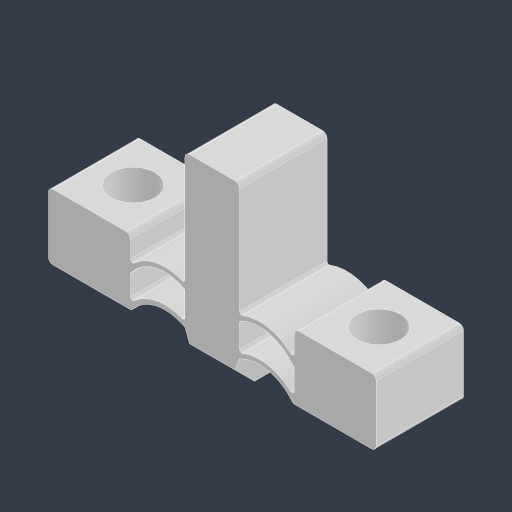
# Autodesk Inventor part: Actuator
Saved by Autodesk Inventor 2023.4 (Build 274418000, 418)
## iProperties
Created: 2024-02-27
Part Number: Actuator
Material: Generic
Document SubType Name: Modeling
Designer: JoaoSilva
Density: 1 g/cm^3
Appearance: Default
Author: JoaoSilva
Autodesk Inventor part; units mm, degrees
ref_plane "YZ Plane" through (0, 0, 0) normal (1, 0, 0) x (0, 1, 0)
ref_plane "XZ Plane" through (0, 0, 0) normal (0, 1, 0) x (-1, 0, 0)
ref_plane "XY Plane" through (0, 0, 0) normal (0, 0, 1) x (1, 0, 0)
sketch "Sketch1" plane through (0, 0, 0) normal (0, 0, 1) x (1, 0, 0)
  line L0 (-2.5, 9) -> (2.5, 9)
  line L1 (2.5, 9) -> (2.5, -9)
  line L2 (2.5, -9) -> (-2.5, -9)
  line L3 (-2.5, -9) -> (-2.5, 9)
  line L4 (-2.5, 9) -> (2.5, -9) construction
  line L5 (2.5, 9) -> (-2.5, -9) construction
  line L6 (-15, 0) -> (-7.5, 0)
  line L7 (-7.5, 0) -> (-7.5, -3)
  line L8 (-7.5, -3) -> (-15, -3)
  line L9 (-15, -3) -> (-15, 0)
  line L10 (7.5, 0) -> (15, 0)
  line L11 (15, 0) -> (15, -3)
  line L12 (15, -3) -> (7.5, -3)
  line L13 (7.5, -3) -> (7.5, 0)
  line L14 (7.5, -3) -> (7.5, -6)
  line L15 (7.5, -6) -> (15, -6)
  line L16 (15, -6) -> (15, -3)
  line L17 (-7.5, -3) -> (-7.5, -6)
  line L18 (-7.5, -6) -> (-15, -6)
  line L19 (-15, -6) -> (-15, -3)
  line L20 (-7.5, -1.5) -> (7.5, -1.5) construction
  line L21 (-1, -9) -> (-2.5, -4.878784)
  line L22 (1, -9) -> (2.5, -4.878784)
  arc A0 (-2.5, -4.678784) -> (-7.5, -5.8) centre (-4.32787, -8.236717) ccw construction
  arc A1 (-2.408606, -4.500887) -> (-7.658606, -5.678164) centre (-4.32787, -8.236717) ccw
  arc A2 (-2.591394, -4.856681) -> (-7.341394, -5.921836) centre (-4.32787, -8.236717) ccw
  arc A3 (-2.591394, -4.856681) -> (-2.408606, -4.500887) centre (-2.5, -4.678784) ccw
  arc A4 (-7.658606, -5.678164) -> (-7.341394, -5.921836) centre (-7.5, -5.8) ccw
  arc A5 (7.5, -5.8) -> (2.5, -4.678784) centre (4.32787, -8.236717) ccw construction
  arc A6 (7.658606, -5.678164) -> (2.408606, -4.500887) centre (4.32787, -8.236717) ccw
  arc A7 (7.341394, -5.921836) -> (2.591394, -4.856681) centre (4.32787, -8.236717) ccw
  arc A8 (7.341394, -5.921836) -> (7.658606, -5.678164) centre (7.5, -5.8) ccw
  arc A9 (2.408606, -4.500887) -> (2.591394, -4.856681) centre (2.5, -4.678784) ccw
  arc A10 (-2.5, -1.678784) -> (-7.5, -2.8) centre (-4.32787, -5.236717) ccw construction
  arc A11 (-2.408606, -1.500887) -> (-7.658606, -2.678164) centre (-4.32787, -5.236717) ccw
  arc A12 (-2.591394, -1.856681) -> (-7.341394, -2.921836) centre (-4.32787, -5.236717) ccw
  arc A13 (-2.591394, -1.856681) -> (-2.408606, -1.500887) centre (-2.5, -1.678784) ccw
  arc A14 (-7.658606, -2.678164) -> (-7.341394, -2.921836) centre (-7.5, -2.8) ccw
  arc A15 (7.5, -2.8) -> (2.5, -1.678784) centre (4.32787, -5.236717) ccw construction
  arc A16 (7.658606, -2.678164) -> (2.408606, -1.500887) centre (4.32787, -5.236717) ccw
  arc A17 (7.341394, -2.921836) -> (2.591394, -1.856681) centre (4.32787, -5.236717) ccw
  arc A18 (7.341394, -2.921836) -> (7.658606, -2.678164) centre (7.5, -2.8) ccw
  arc A19 (2.408606, -1.500887) -> (2.591394, -1.856681) centre (2.5, -1.678784) ccw
  point P0 (0, 0)
  point P1 (0, -1.5)
  point P2 (-7.5, -5.483975)
  point P3 (-2.5, -1.878784)
  point P4 (-2.5, -4.45533)
  point P5 (7.5, -5.483975)
  point P6 (2.5, -4.45533)
  point P7 (2.5, -1.878784)
  point P8 (7.5, -2.483975)
  point P9 (2.5, -1.45533)
  point P10 (-2.5, -1.45533)
  point P11 (-7.5, -2.483975)
  dimension "d0" = 5
  dimension "d1" = 18
  dimension "d2" = 30
  dimension "d3" = 3
  dimension "d4" = 3
  dimension "d5" = 5
  dimension "d8" = 9
  dimension "d9" = 3
  dimension "d10" = 2
  dimension "d11" = 20
  dimension "d12" = 0.4
  dimension "d13" = 4
  dimension "d14" = 3
  constraints: 46 end point, 42 point on circle, 20 centre point, 18 tangent, 14 point on line, 7 perpendicular, 6 equal radius, 6 parallel, 5 midpoint, 3 collinear, 3 equal length, 3 horizontal, 3 vertical alignment, 2 horizontal alignment, 2 vertical
  measures "d0" distance of L0.start L0.end
  measures "d1" distance of L0.end L1.end
  measures "d2" distance between parallel lines of L11 L9
  measures "d3" distance between parallel lines of L2 L18
  measures "d4" distance between parallel lines of L2 L15
  measures "d5" distance between parallel lines of L3 L17
  measures "d8" distance between parallel lines of L2 L6
  measures "d9" distance of L8.end L6.start
  measures "d10" distance of L22.start L21.start
  measures "d11" angle of L3 L21
  measures "d12" radial gap between concentric circles of A1 A2
  measures "d13" radius of A0
  measures "d14" distance of A0.centre A10.centre
sketch "Sketch1 outline for Extrusion1" plane through (0, 0, 0) normal (0, 0, 1) x (1, 0, 0)
  arc A0 (-7.5, -6) -> (-7.341394, -5.921836) centre (-7.5, -5.8) ccw
  line L0 (-15, -6) -> (-7.5, -6)
  arc A1 (-7.341394, -5.921836) -> (-2.591394, -4.856681) centre (-4.32787, -8.236717) cw
  line L1 (-15, -3) -> (-15, -6)
  arc A2 (-2.591394, -4.856681) -> (-2.5, -4.878784) centre (-2.5, -4.678784) ccw
  line L2 (-15, 0) -> (-15, -3)
  line L3 (-2.5, -4.878784) -> (-1, -9)
  line L4 (-7.5, 0) -> (-15, 0)
  line L5 (-1, -9) -> (1, -9)
  line L6 (-7.5, -2.483975) -> (-7.5, 0)
  line L7 (1, -9) -> (2.5, -4.878784)
  arc A3 (-2.5, -1.45533) -> (-7.5, -2.483975) centre (-4.32787, -5.236717) ccw
  arc A4 (2.5, -4.878784) -> (2.591394, -4.856681) centre (2.5, -4.678784) ccw
  line L8 (-2.5, 9) -> (-2.5, -1.45533)
  arc A5 (2.591394, -4.856681) -> (7.341394, -5.921836) centre (4.32787, -8.236717) cw
  line L9 (2.5, 9) -> (-2.5, 9)
  arc A6 (7.341394, -5.921836) -> (7.5, -6) centre (7.5, -5.8) ccw
  line L10 (2.5, -1.45533) -> (2.5, 9)
  line L11 (7.5, -6) -> (15, -6)
  arc A7 (7.5, -2.483975) -> (2.5, -1.45533) centre (4.32787, -5.236717) ccw
  line L12 (15, -6) -> (15, -3)
  line L13 (7.5, 0) -> (7.5, -2.483975)
  line L14 (15, -3) -> (15, 0)
  line L15 (15, 0) -> (7.5, 0)
  line L16 (-7.5, -5.483975) -> (-7.5, -3)
  arc A8 (-2.5, -4.45533) -> (-7.5, -5.483975) centre (-4.32787, -8.236717) ccw
  line L17 (-2.5, -1.878784) -> (-2.5, -4.45533)
  arc A9 (-2.591394, -1.856681) -> (-2.5, -1.878784) centre (-2.5, -1.678784) ccw
  arc A10 (-7.341394, -2.921836) -> (-2.591394, -1.856681) centre (-4.32787, -5.236717) cw
  arc A11 (-7.5, -3) -> (-7.341394, -2.921836) centre (-7.5, -2.8) ccw
  arc A12 (7.5, -5.483975) -> (2.5, -4.45533) centre (4.32787, -8.236717) ccw
  line L18 (7.5, -3) -> (7.5, -5.483975)
  arc A13 (7.341394, -2.921836) -> (7.5, -3) centre (7.5, -2.8) ccw
  arc A14 (2.591394, -1.856681) -> (7.341394, -2.921836) centre (4.32787, -5.236717) cw
  arc A15 (2.5, -1.878784) -> (2.591394, -1.856681) centre (2.5, -1.678784) ccw
  line L19 (2.5, -4.45533) -> (2.5, -1.878784)
extrude "Extrusion1" add sketch "Sketch1 outline for Extrusion1" along normal blind 8
chamfer "Chamfer1" distance 3 angle 45 1 edges at (0, -9, 0) measured on face at (-0.3333, -9, 2.6667)
chamfer "Chamfer2" distance 3 angle 45 1 edges at (0, -9, 8) measured on face at (-0.3333, -9, 4.6667)
fillet "Fillet1" radius 0.2 14 edges at (-7.5, -2.484, 4) (-7.5, -3, 4) (-7.5, -5.484, 4) (-2.5, -4.8788, 4) (-2.5, -4.4553, 4) (-2.5, -1.8788, 4) (-2.5, -1.4553, 4) (2.5, -1.4553, 4) (2.5, -1.8788, 4) (2.5, -4.4553, 4) (2.5, -4.8788, 4) (7.5, -5.484, 4) (7.5, -3, 4) (7.5, -2.484, 4)
fillet "Fillet2" radius 0.4 12 edges at (-15, 0, 4) (-15, -3, 4) (15, -3, 4) (15, 0, 4) (7.5, 0, 4) (15, -6, 4) (-15, -6, 4) (-7.5, 0, 4) (-2.5, 9, 4) (2.5, 9, 4) (-1, -9, 4) (1, -9, 4)
sketch "Sketch3" plane through (-14.6, 0, 0) normal (0, 1, 0) x (1, 0, 0)
  line L0 (3.35, -4) -> (25.85, -4) construction
  line L1 (16.7, 0) -> (12.5, 0) projected
  line L2 (29.2, 0) -> (29.2, -8) projected
  line L3 (6.7, -8) -> (0, -8) projected
  point P0 (14.6, 0)
  point P1 (14.6, -4)
  point P2 (14.6, 0)
  point P3 (29.2, -4)
  point P4 (3.35, -8)
  constraints: 4 midpoint, 2 end point, 2 vertical alignment, 1 horizontal, 1 horizontal alignment
hole "Hole2" at (-11.25, 0, 4) at (11.25, 0, 4) direction (0, -1, 0) diameter 4 end through all
equation "\"d4\" = d3"
body "Solid1"
